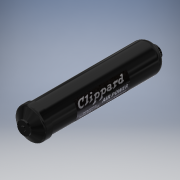
# Autodesk Inventor part: AVT-PP-35
Saved by Autodesk Inventor 2018.2 (Build 222227000, 227)
## iProperties
Category: Loose
Company: Autodesk Inc.
Created: 2017-12-10
Part Number: AVT-PP-35
Material: Steel
Document SubType Name: Modeling
Designer: Autodesk Inc.
Density: 7.85 g/cm^3
Appearance: Smooth - Black
Catalog Web Link: http://www.clippard.com/downloads/PDF_Documents/Clippard%20Full%20Line%20Catalog/Clippard%20Catalog%20by%20Page%20Number/Air%20Cylinders/Page%20065.pdf
Vendor: Clippard
Author: Autodesk Inc.
Keywords: Gray Tote
Autodesk Inventor part; units mm, degrees
ref_plane "XZ Plane" through (0, 0, 0) normal (0, 1, 0) x (-1, 0, 0)
ref_plane "XY Plane" through (0, 0, 0) normal (0, 0, 1) x (1, 0, 0)
sketch "Sketch1" plane through (0, 0, 0) normal (0, 1, 0) x (-1, 0, 0)
  line L0 (0, 0) -> (0, -394.9191)
  line L1 (0, 0) -> (32.512, 0)
  line L2 (32.512, 0) -> (32.512, -265.6586)
  line L3 (32.512, -265.6586) -> (0, -265.6586)
  dimension "d0" = 32.512
  dimension "d1" = 265.6586
  constraints: 8 end point, 2 perpendicular, 1 horizontal, 1 point on line, 1 vertical
  measures "d0" distance of L0.start L1.end
  measures "d1" distance of L1.end L2.end
revolve "Revolution1" add sketch "Sketch1" angle 360 about axis through (0, 0, 0) along (0, 0, -1)
fillet "Fillet1" radius 19.05 1 edges at (32.512, 0, -265.6586)
sketch "Sketch2" plane through (0, 0, 0) normal (1, 0, 0) x (0, 1, 0)
  line L0 (0, 0) -> (35.306, 0)
  line L1 (-32.512, 0) -> (32.512, 0) projected
  line L2 (35.306, 0) -> (35.306, 19.05)
  line L3 (35.306, 19.05) -> (0, 19.05)
  line L4 (0, 19.05) -> (0, 0)
  dimension "d4" = 35.306
  dimension "d5" = 19.05
  constraints: 8 end point, 2 perpendicular, 1 collinear, 1 vertical
  measures "d4" distance of L0.start L0.end
  measures "d5" distance of L0.end L2.end
revolve "Revolution2" add sketch "Sketch2" angle 360 about axis through (0, 0, 19.05) along (0, 0, -1)
fillet "Fillet2" radius 6.35 1 edges at (0, -35.306, 19.05)
sketch "Sketch3" plane through (0, 0, 0) normal (1, 0, 0) x (0, 1, 0)
  arc A0 (35.306, 12.7) -> (28.956, 19.05) centre (28.956, 12.7) ccw projected
  line L0 (32.267, 18.1184) -> (14.7581, 28.8176)
  line L1 (14.7581, 28.8176) -> (0, 28.8176)
  line L2 (0, 28.8176) -> (0, 19.05)
  line L3 (-28.956, 19.05) -> (28.956, 19.05) projected
  point P0 (0, 0)
  constraints: 6 end point, 1 horizontal, 1 midpoint, 1 point on circle, 1 tangent
revolve "Revolution3" add sketch "Sketch3" angle 360 about axis through (0, 0, 28.8176) along (0, 0, -1)
sketch "Sketch4" plane through (0, 0, 28.8176) normal (0, 0, 1) x (1, 0, 0)
  circle A0 centre (0, 0) radius 14.7581 projected
extrude "Extrusion1" add sketch "Sketch4" along normal blind 3.6576
sketch "Sketch5" plane through (0, 0, -265.6586) normal (0, 0, -1) x (-1, 0, 0)
  circle A0 centre (0, 0) radius 13.462 projected
extrude "Extrusion2" add sketch "Sketch5" along normal blind 8.1788
sketch "Sketch6" plane through (0, 0, 32.4752) normal (0, 0, 1) x (1, 0, 0)
  circle A0 centre (0, 0) radius 14.7581 projected
  circle A1 centre (0, 0) radius 5.1761
  constraints: 1 centre point, 1 coincident
extrude "Extrusion3" add sketch "Sketch6" along normal blind 2.54 contours A1
sketch "Sketch7" plane through (0, 0, -273.8374) normal (0, 0, -1) x (-1, 0, 0)
  circle A0 centre (0, 0) radius 5.1761 projected
extrude "Extrusion4" add sketch "Sketch7" along normal blind 2.54
ref_plane "Work Plane1" through (32.512, 0, -132.8293) normal (1, 0, 0) x (0, 1, 0)
sketch "Sketch8" plane through (32.512, 0, -132.8293) normal (1, 0, 0) x (0, 1, 0)
  line L0 (25.1558, 74.2307) -> (25.1558, -47.9866) construction
  line L1 (25.1558, -47.9866) -> (-21.6706, -47.9866) construction
  line L2 (-21.6706, -47.9866) -> (-21.6706, 74.2307) construction
  line L3 (-21.6706, 74.2307) -> (25.1558, 74.2307) construction
  point P0 (0, 132.8293)
  constraints: 1 vertical, 2 other
decal "Decal1"
body "Solid1"
